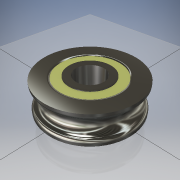
# Autodesk Inventor part: idler bearing
Saved by Autodesk Inventor 2016 SP1 (Build 200210100, 210)
## iProperties
Created: 2015-12-27
Part Number: idler bearing
Material: Generic
Document SubType Name: Modeling
Designer: Dirk Alferink
Density: 1 g/cm^3
Appearance: Silver
Author: Dirk Alferink
Autodesk Inventor part; units mm, degrees
ref_plane "YZ Plane" through (0, 0, 0) normal (1, 0, 0) x (0, 1, 0)
ref_plane "XZ Plane" through (0, 0, 0) normal (0, 1, 0) x (-1, 0, 0)
sketch "Sketch1" plane through (0, 0, 0) normal (0, 0, 1) x (1, 0, 0)
  line L0 (6.5, 2) -> (2, 2)
  line L1 (2, 2) -> (2, 0)
  line L2 (0, 0) -> (0, 12.2803)
  circle A0 centre (6.5, 0) radius 1.25
  line L3 (6.5, 1.25) -> (6.5, 2)
  line L4 (5.25, 0) -> (2, 0)
  dimension "d0" = 4.5
  dimension "d2" = 2
  dimension "d3" = 2.5
  constraints: 10 end point, 2 point on circle, 2 vertical, 1 centre point, 1 perpendicular, 1 vertical alignment
  measures "d0" distance of L0.end L0.start
  measures "d2" distance from line of L2.start L1
  measures "d3" diameter of A0
revolve "Revolution1" add sketch "Sketch1" angle 360 about axis through (0, 0, 0) along (0, 1, 0) contours L3 A0 L4 L1 L0
ref_plane "Work Plane1" through (0, 0, 0) normal (0, -1, 0) x (1, 0, 0)
sketch "Sketch2" plane through (0, 2, 0) normal (0, 1, 0) x (1, 0, 0)
  circle A0 centre (0, 0) radius 3
  circle A1 centre (0, 0) radius 4.25
  dimension "d6" = 6
  dimension "d7" = 8.5
  constraints: 2 centre point, 2 coincident
  measures "d6" diameter of A0
  measures "d7" diameter of A1
extrude "Extrusion1" cut sketch "Sketch2" against normal blind 0.1
fillet "Fillet1" radius 0.5 1 edges at (-4.25, 2, 0)
mirror "Mirror1" about plane through (0, 0, 0) normal (0, -1, 0) of "Revolution1", "Extrusion1", "Fillet1"
fillet "Fillet2" radius 0.5 2 edges at (-6.5, -1.25, 0) (-6.5, 1.25, 0)
body "Solid1"
